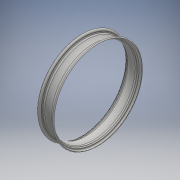
# Autodesk Inventor part: Rim
Saved by Autodesk Inventor 2016 (Build 200138000, 138)
## iProperties
Created: 2016-01-10
Part Number: Rim
Material: Générique
Document SubType Name: Modeling
Designer: Cyril
Density: 1 g/cm^3
Appearance: Par défaut
Author: Cyril
Autodesk Inventor part; units mm, degrees
ref_plane "YZ Plane" through (0, 0, 0) normal (1, 0, 0) x (0, 1, 0)
ref_plane "XZ Plane" through (0, 0, 0) normal (0, 1, 0) x (-1, 0, 0)
ref_plane "XY Plane" through (0, 0, 0) normal (0, 0, 1) x (1, 0, 0)
sketch "Esquisse1" plane through (0, 0, 0) normal (0, 0, 1) x (1, 0, 0)
  arc A0 (-16.1737, 200.4256) -> (0, 194.8) centre (0, 220.8625) ccw
  arc A1 (-16.1737, 200.4256) -> (-23, 202.8) centre (-23, 191.8) ccw
  line L0 (-23, 202.8) -> (-25.5, 202.8)
  arc A2 (-27.5, 204.8) -> (-25.5, 202.8) centre (-25.5, 204.8) ccw
  line L1 (-27.5, 204.8) -> (-27.5, 207.3)
  arc A3 (-27.5, 207.3) -> (-35.5, 215.3) centre (-35.5, 207.3) ccw
  arc A4 (-35.5, 215.3) -> (-39.9777, 211.7745) centre (-35.5, 210.6937) ccw
  line L2 (-35.5, 207.3) -> (-35.5, 215.3) construction
  line L3 (0, -44.1725) -> (0, 265.035) construction
  arc A5 (0, 194.8) -> (16.1737, 200.4256) centre (0, 220.8625) ccw
  arc A6 (23, 202.8) -> (16.1737, 200.4256) centre (23, 191.8) ccw
  line L4 (23, 202.8) -> (25.5, 202.8)
  arc A7 (25.5, 202.8) -> (27.5, 204.8) centre (25.5, 204.8) ccw
  line L5 (27.5, 204.8) -> (27.5, 207.3)
  arc A8 (35.5, 215.3) -> (27.5, 207.3) centre (35.5, 207.3) ccw
  arc A9 (39.9777, 211.7745) -> (35.5, 215.3) centre (35.5, 210.6937) ccw
  line L6 (35.5, 207.3) -> (35.5, 215.3) construction
  arc A10 (-35.5, 213.7) -> (-38.4223, 211.3991) centre (-35.5, 210.6937) ccw
  arc A11 (-29.1, 207.3) -> (-35.5, 213.7) centre (-35.5, 207.3) ccw
  line L7 (-29.1, 207.3) -> (-29.1, 204.8)
  arc A12 (-29.1, 204.8) -> (-25.5, 201.2) centre (-25.5, 204.8) ccw
  line L8 (-25.5, 201.2) -> (-23, 201.2)
  arc A13 (-17.1666, 199.171) -> (-23, 201.2) centre (-23, 191.8) ccw
  arc A14 (-17.1666, 199.171) -> (11.0067, 195.484) centre (0, 220.8625) ccw
  arc A15 (11.0067, 195.484) -> (17.1666, 199.171) centre (0, 220.8625) ccw
  arc A16 (23, 201.2) -> (17.1666, 199.171) centre (23, 191.8) ccw
  line L9 (23, 201.2) -> (25.5, 201.2)
  arc A17 (25.5, 201.2) -> (29.1, 204.8) centre (25.5, 204.8) ccw
  line L10 (29.1, 204.8) -> (29.1, 207.3)
  arc A18 (35.5, 213.7) -> (29.1, 207.3) centre (35.5, 207.3) ccw
  arc A19 (38.4223, 211.3991) -> (35.5, 213.7) centre (35.5, 210.6937) ccw
  arc A20 (-39.9777, 211.7745) -> (-38.4223, 211.3991) centre (-39.2, 211.5868) ccw
  arc A21 (38.4223, 211.3991) -> (39.9777, 211.7745) centre (39.2, 211.5868) ccw
  line L11 (-56.8237, 0) -> (56.8237, 0) projected
  point P0 (0, 0)
  dimension "d0" = 202.8
  dimension "d3" = 2
  dimension "d5" = 8
  dimension "d6" = 4.5
  dimension "d8" = 8
  dimension "d13" = 4.5
  dimension "d16" = 1.6
  dimension "d19" = 12.5
  dimension "d20" = 12.5
  dimension "d21" = 4.6063
  dimension "d23" = 55
  dimension "d24" = 11
  dimension "d25" = 26.0625
  constraints: 45 point on circle, 22 centre point, 20 end point, 13 symmetric about line, 8 tangent, 2 vertical, 2 vertical alignment, 1 horizontal, 19 other
  measures "d0" distance from line of point (0, 0) L0
  measures "d3" radius of A2
  measures "d5" radius of A3
  measures "d6" distance from line of L1 A1.centre
  measures "d8" distance from line of A0.end L0
  measures "d13" distance from line of L0 L2.start
  measures "d16" radial gap between concentric circles of A3 A11
  measures "d20" distance from line of L0 L2.end
  measures "d21" radius of A4
  measures "d23" distance between parallel lines of L5 L1
  measures "d24" radius of A1
  measures "d25" radius of A0
revolve "Révolution1" add sketch "Esquisse1" angle 360 about axis through (-10, 0, 0) along (1, 0, 0)
